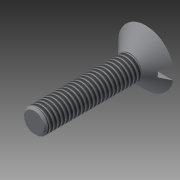
# Autodesk Inventor part: 载板连接销固定螺丝
Saved by Autodesk Inventor 2015 (Build 190159000, 159)
## iProperties
Created: 2017-05-02
Part Number: 载板连接销固定螺丝
Material: 常规
Document SubType Name: Modeling
Designer: Administrator
Density: 1 g/cm^3
Appearance: 默认
Author: Administrator
Autodesk Inventor part; units mm, degrees
ref_plane "XZ Plane" through (0, 0, 0) normal (0, 1, 0) x (-1, 0, 0)
ref_plane "XY Plane" through (0, 0, 0) normal (0, 0, 1) x (1, 0, 0)
sketch "草图1" plane through (0, 0, 0) normal (0, 0, 1) x (1, 0, 0)
  line L0 (-3.5, 2) -> (0, 2)
  line L1 (0, 2) -> (0, 0)
  line L2 (0, 0) -> (-1.5, 0)
  line L3 (-1.5, 0) -> (-3.5, 2)
  line L4 (0, -0.4) -> (0, 2.4) projected
  dimension "d0" = 3.5
  dimension "d1" = 2
  dimension "d2" = 1.5
  constraints: 8 end point, 2 perpendicular, 1 horizontal
  measures "d0" distance of L0.start L0.end
  measures "d1" distance of L0.end L1.end
  measures "d2" distance of L1.end L2.end
revolve "旋转1" add sketch "草图1" angle 360 about axis through (0, -10, 0) along (0, 1, 0)
sketch "草图2" plane through (0, 0, 0) normal (0, -1, 0) x (1, 0, 0)
  circle A0 centre (0, 0) radius 1.5
  dimension "d4" = 3
  constraints: 1 centre point, 1 coincident
  measures "d4" diameter of A0
extrude "拉伸1" add sketch "草图2" along normal blind 12
chamfer "倒角1" distance 0.25 angle 45 1 edges at (-1.5, -12, 0)
thread "螺纹1" size "M3x0.5" class "6g" standard "ANSI Metric M Profile" full length
ref_plane "工作平面1" through (3.5, 0, 0) normal (1, 0, 0) x (0, 1, 0)
sketch "草图3" plane through (3.5, 0, 0) normal (1, 0, 0) x (0, 1, 0)
  line L0 (2, -0.75) -> (1, -0.4)
  line L1 (1, -0.4) -> (1, 0.4)
  line L2 (2, -3.5) -> (2, 3.5) projected
  line L3 (1, 0.4) -> (2, 0.75)
  line L4 (2, 0.75) -> (2, -0.75)
  point P0 (0, 0)
  point P1 (2, 0)
  dimension "d13" = 1
  dimension "d14" = 0.8
  dimension "d15" = 1.5
  constraints: 8 end point, 2 midpoint, 2 parallel, 1 equal length
  measures "d13" distance between parallel lines of L2 L1
  measures "d14" distance of L0.end L1.end
  measures "d15" distance of L3.end L0.start
extrude "拉伸2" cut sketch "草图3" against normal blind 7
